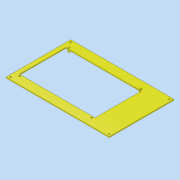
# Autodesk Inventor part: touchscreen_lid
Saved by Autodesk Inventor 2022 (Build 260153000, 153)
## iProperties
Created: 2020-11-06
Part Number: touchscreen_lid
Material: Generic
Document SubType Name: Modeling
Designer: nnico
Density: 1 g/cm^3
Appearance: Yellow
Author: nnico
Autodesk Inventor part; units mm, degrees
ref_plane "YZ Plane" through (0, 0, 0) normal (1, 0, 0) x (0, 1, 0)
ref_plane "XZ Plane" through (0, 0, 0) normal (0, 1, 0) x (-1, 0, 0)
ref_plane "XY Plane" through (0, 0, 0) normal (0, 0, 1) x (1, 0, 0)
sketch "Sketch1" plane through (0, 0, 0) normal (0, 1, 0) x (-1, 0, 0)
  line L0 (103.4541, -70.75) -> (-122.0459, -70.75)
  line L1 (-122.0459, -70.75) -> (-122.0459, 70.75)
  line L2 (-122.0459, 70.75) -> (103.4541, 70.75)
  line L3 (103.4541, 70.75) -> (103.4541, -70.75)
  line L4 (94.4541, -50.75) -> (-71.0459, -50.75)
  line L5 (-71.0459, -50.75) -> (-71.0459, 50.75)
  line L6 (-71.0459, 50.75) -> (94.4541, 50.75)
  line L7 (94.4541, 50.75) -> (94.4541, -50.75)
  line L8 (11.7041, -50.75) -> (11.7041, 50.75) construction
  line L9 (94.4541, 0) -> (-71.0459, 0) construction
  circle A0 centre (98.4541, -65.75) radius 1.75
  line L10 (103.4541, -70.75) -> (98.4541, -70.75) construction
  line L11 (98.4541, -70.75) -> (98.4541, -65.75) construction
  line L12 (98.4541, -65.75) -> (103.4541, -65.75) construction
  line L13 (103.4541, -65.75) -> (103.4541, -70.75) construction
  circle A1 centre (-117.0459, -65.75) radius 1.75
  circle A2 centre (98.4541, 65.75) radius 1.75
  circle A3 centre (-117.0459, 65.75) radius 1.75
  dimension "d0" = 101.5
  dimension "d1" = 165.5
  dimension "d3" = 20
  dimension "d4" = 3.5
  dimension "d5" = 5
  dimension "d6" = 5
  dimension "d14" = 225.5
  dimension "d16" = 9
  dimension "d21" = 5
  dimension "d22" = 5
  constraints: 28 end point, 6 parallel, 4 centre point, 4 midpoint, 3 horizontal, 3 perpendicular, 1 coincident, 1 symmetric about line, 3 other
  measures "d0" distance of L6.end L4.start
  measures "d1" distance of L4.start L4.end
  measures "d3" distance from line of L0 L4.end
  measures "d4" diameter of A0
  measures "d5" distance of L11.end L12.end
  measures "d6" distance of L10.end L11.end
  measures "d14" distance of L0.start L0.end
  measures "d16" distance from line of L3 L4.start
  measures "d21" distance from line of L1 A1.centre
  measures "d22" distance from line of L0 A1.centre
extrude "Extrusion1" add sketch "Sketch1" along normal blind 2
sketch "Sketch2" plane through (0, 2, 0) normal (0, 1, 0) x (1, 0, 0)
  line L0 (122.0459, 70.75) -> (-103.4541, 70.75) construction
  line L1 (-103.4541, -70.75) -> (122.0459, -70.75) construction
  line L2 (-103.4541, 70.75) -> (-103.4541, -70.75) construction
  line L3 (-103.4541, 0) -> (122.0459, 0) construction
  line L4 (122.0459, -70.75) -> (122.0459, 70.75) construction
  circle A0 centre (-90.3171, 54.112) radius 1.75
  circle A1 centre (66.9089, 54.112) radius 1.75
  circle A2 centre (-90.3171, -54.112) radius 1.75
  circle A3 centre (66.9089, -54.112) radius 1.75
  line L5 (71.0459, -50.75) -> (-94.4541, -50.75) construction
  line L6 (-11.7041, -50.75) -> (-11.7041, 50.75) construction
  line L7 (-94.4541, 50.75) -> (71.0459, 50.75) construction
  point P0 (0, 0)
  dimension "d9" = 3.5
  dimension "d11" = 108.224
  dimension "d17" = 157.226
  constraints: 4 centre point, 4 end point, 4 midpoint, 3 symmetric about line, 2 other
  measures "d9" diameter of A0
  measures "d11" diameter of A0.centre L3
  measures "d17" distance of A1.centre A0.centre
extrude "Extrusion2" cut sketch "Sketch2" against normal up to next
sketch "Sketch3" plane through (0, 2, 0) normal (0, 1, 0) x (1, 0, 0)
  circle A0 centre (-90.3171, 54.112) radius 1.75 projected
  circle A1 centre (-90.3171, 54.112) radius 3
  line L0 (-94.4541, 50.75) -> (71.0459, 50.75) construction
  line L1 (-11.7041, 50.75) -> (-11.7041, -50.75) construction
  line L2 (71.0459, -50.75) -> (-94.4541, -50.75) construction
  line L3 (-94.4541, -50.75) -> (-94.4541, 50.75) construction
  line L4 (-94.4541, 0) -> (71.0459, 0) construction
  line L5 (71.0459, -50.75) -> (71.0459, 50.75) construction
  circle A2 centre (66.9089, 54.112) radius 3
  circle A3 centre (-90.3171, -54.112) radius 3
  circle A4 centre (66.9089, -54.112) radius 3
  circle A5 centre (-90.3171, -54.112) radius 1.75 projected
  circle A6 centre (66.9089, -54.112) radius 1.75 projected
  circle A7 centre (66.9089, 54.112) radius 1.75 projected
  point P0 (0, 0)
  dimension "d18" = 6
  constraints: 4 centre point, 4 end point, 4 midpoint, 3 symmetric about line, 1 coincident, 3 other
  measures "d18" diameter of A1
extrude "Extrusion3" add sketch "Sketch3" against normal blind 7
body "Solid1"
